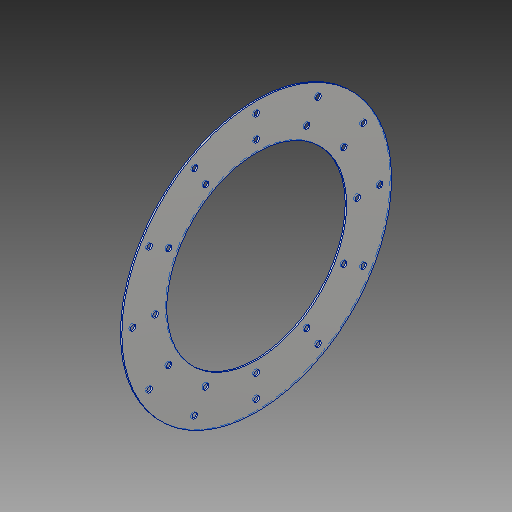
# Autodesk Inventor part: Wall
Saved by Autodesk Inventor 2019 (Build 230136000, 136)
## iProperties
Created: 2017-04-20
Part Number: Wall
Material: Aluminum 6061
Document SubType Name: Modeling
Designer: Adhikara
Density: 2.7 g/cm^3
Appearance: Aluminum - Flat
Mass: 170.492 g
Surface Area: 828.467 cm^2
Volume: 63.1453 cm^3
Author: Adhikara
Autodesk Inventor part; units mm, degrees
ref_plane "YZ Plane" through (0, 0, 0) normal (1, 0, 0) x (0, 1, 0)
ref_plane "XZ Plane" through (0, 0, 0) normal (0, 1, 0) x (-1, 0, 0)
ref_plane "XY Plane" through (0, 0, 0) normal (0, 0, 1) x (1, 0, 0)
sketch "Sketch1" plane through (0, 0, 0) normal (1, 0, 0) x (0, 1, 0)
  circle A0 centre (0, 0) radius 152.4
  line L0 (-213.36, 0) -> (213.36, 0) construction
  line L1 (0, -213.36) -> (0, 213.36) construction
  circle A1 centre (0, 139.7) radius 3.175
  circle A2 centre (0, 114.3) radius 3.175
  circle A3 centre (-69.85, 120.9837) radius 3.175
  circle A4 centre (-57.15, 98.9867) radius 3.175
  circle A5 centre (-120.9837, 69.85) radius 3.175
  circle A6 centre (-98.9867, 57.15) radius 3.175
  circle A7 centre (-139.7, 0) radius 3.175
  circle A8 centre (-114.3, 0) radius 3.175
  circle A9 centre (-120.9837, -69.85) radius 3.175
  circle A10 centre (-98.9867, -57.15) radius 3.175
  circle A11 centre (-69.85, -120.9837) radius 3.175
  circle A12 centre (-57.15, -98.9867) radius 3.175
  circle A13 centre (0, -139.7) radius 3.175
  circle A14 centre (0, -114.3) radius 3.175
  circle A15 centre (69.85, -120.9837) radius 3.175
  circle A16 centre (57.15, -98.9867) radius 3.175
  circle A17 centre (120.9837, -69.85) radius 3.175
  circle A18 centre (98.9867, -57.15) radius 3.175
  circle A19 centre (139.7, 0) radius 3.175
  circle A20 centre (114.3, 0) radius 3.175
  circle A21 centre (120.9837, 69.85) radius 3.175
  circle A22 centre (98.9867, 57.15) radius 3.175
  circle A23 centre (69.85, 120.9837) radius 3.175
  circle A24 centre (57.15, 98.9867) radius 3.175
  point P0 (0, 152.4)
  dimension "d0" = 304.8
  dimension "d1" = 12.7
  dimension "d2" = 25.4
  dimension "d3" = 6.35
  dimension "d6" = 360
  constraints: 24 centre point, 3 point on line, 1 coincident, 1 equal radius, 1 vertical alignment, 51 other
  measures "d1" distance of A1.centre point (0, 152.4)
  measures "d2" distance of A1.centre A2.centre
  measures "d3" diameter of A2
extrude "Extrusion1" add sketch "Sketch1" along normal blind 1.5875
sketch "Sketch2" plane through (1.5875, 0, 0) normal (1, 0, 0) x (0, 0, -1)
  circle A0 centre (0, 0) radius 101.6
  dimension "d10" = 203.2
  constraints: 1 centre point, 1 coincident
  measures "d10" diameter of A0
extrude "Extrusion2" cut sketch "Sketch2" against normal through all
body "Solid1"
